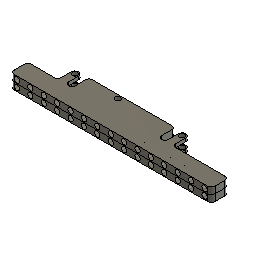
_Bottom Attatchment.85361469-475e-472e-92d3-0b1b0a94a3bd (Autodesk Fusion 360 design; units mm, degrees)
Autodesk Fusion 360 part; units mm, degrees
sketch "Sketch1" plane through (0, 0, 0) normal (0, 1, 0) x (1, 0, 0)
  circle A0 centre (25.25, 23) radius 2
  circle A1 centre (57.25, 23) radius 2
  circle A2 centre (105.25, 23) radius 2
  circle A3 centre (25.25, 23) radius 2.75
  circle A4 centre (57.25, 23) radius 2.75
  circle A5 centre (105.25, 23) radius 2.75
  line L0 (28, 23) -> (28, 13)
  line L1 (28, 13) -> (33, 13)
  line L2 (33, 13) -> (33, 25.75)
  line L3 (33, 25.75) -> (97.5, 25.75)
  line L4 (97.5, 25.75) -> (97.5, 13)
  line L5 (97.5, 13) -> (102.5, 13)
  line L6 (102.5, 13) -> (102.5, 23)
  line L7 (108, 23) -> (108, 13)
  line L8 (108, 13) -> (150, 13)
  line L9 (150, 13) -> (150, 0)
  line L10 (150, 0) -> (0, 0)
  line L11 (0, 0) -> (0, 13)
  line L12 (0, 13) -> (22.5, 13)
  line L13 (22.5, 13) -> (22.5, 23)
  line L14 (25.25, 25.75) -> (15.4724, 25.75)
  line L15 (105.25, 25.75) -> (113, 25.75)
  line L16 (108, 13) -> (102.5, 13)
  line L17 (28, 13) -> (22.5, 13)
  line L18 (33, 0) -> (97.5, 0) construction
  line L19 (97.5, 0) -> (97.5, 13) construction
  line L20 (97.5, 13) -> (33, 13) construction
  line L21 (33, 13) -> (33, 0) construction
  dimension "d1" = 4
  dimension "d2" = 5.5
  dimension "d3" = 32
  dimension "d4" = 80
  dimension "d5" = 10
  dimension "d6" = 5
  dimension "d7" = 23
  dimension "d8" = 22.5
  dimension "d9" = 42
  dimension "d10" = 10
  dimension "d33" = 150
  constraint equal A0 A1
  constraint equal A1 A2
  constraint concentric A0 A3
  constraint concentric A1 A4
  constraint concentric A2 A5
  constraint equal A4 A5
  constraint equal A3 A4
  constraint coincident A3 L0.start
  constraint vertical L0
  constraint perpendicular L0 L1
  constraint perpendicular L1 L2
  constraint perpendicular L2 L3
  constraint perpendicular L3 L4
  constraint perpendicular L2 L5
  constraint coincident A5 L6.end
  constraint tangent A5 L6
  constraint coincident A5 L7.start
  constraint parallel L6 L7
  constraint perpendicular L8 L9
  constraint coincident L10.end L11.start
  constraint perpendicular L10 L11
  constraint perpendicular L9 L12
  constraint coincident A3 L13.end
  constraint tangent A3 L13
  constraint horizontal L10
  constraint horizontal L12
  constraint vertical L13
  constraint tangent A4 L3
  constraint coincident A3 L14.start
  constraint horizontal L14
  constraint coincident A5 L15.start
  constraint horizontal L15
  constraint tangent A5 L15
  constraint tangent A3 L14
  constraint collinear L3 L14
  constraint collinear L3 L15
  constraint vertical L6
  constraint equal L7 L13
  constraint equal L1 L5
  constraint equal L2 L4
  constraint equal L6 L7
  constraint tangent A5 L7
  constraint tangent A3 L0
  constraint coincident L10
  constraint coincident L1.end
  constraint collinear L4 L19
  measures "d1" diameter of A0
  measures "d2" diameter of A3
  measures "d3" distance of A0.centre A1.centre
  measures "d4" distance of A0.centre A2.centre
  measures "d5" distance of L7.start L7.end
  measures "d6" distance of L4.end L5.end
  measures "d7" distance of A0.centre L10
  measures "d8" distance of L11.end L12.end
  measures "d9" distance of L7.end L8.end
  measures "d33" distance of L9.end L10.end
extrude "Extrude1" add sketch "Sketch1" along normal blind 5 contours A4 | L1 L2 L3 L4 L5 L8 L9 L10 L11 L12 L16 L17 makes body 1
extrude "Extrude2" add sketch "Sketch1" along normal blind 5 and the other way blind -2.5 contours A3 | A3 L0 L13 L17 | A5 L6 L7 L16 | A5 bodies 1
fillet "Fillet1" radius 2.5 8 edges at (33, 2.5, -25.75) (97.5, 2.5, -25.75) (102.5, 3.75, -13) (97.5, 2.5, -13) (108, 3.75, -13) (33, 2.5, -13) (28, 3.75, -13) (22.5, 3.75, -13) on bodies 1
fillet "Fillet1" radius 3 4 edges at (0, 2.5, -13) (0, 2.5, 0) (150, 2.5, 0) (150, 2.5, -13) on bodies 1
sketch "Sketch2" plane through (0, 0, 0) normal (0, 0, 1) x (1, 0, 0)
  line L0 (147, 0) -> (147, 5)
  line L1 (147, 5) -> (3, 5)
  line L2 (3, 5) -> (3, 0)
  line L3 (3, 0) -> (147, 0)
  circle A0 centre (5, 2.5) radius 1.95
  line L4 (0, 5) -> (0, 0)
  line L5 (5, 2.5) -> (3, 2.5)
  dimension "d25" = 5
  dimension "d26" = 3.9
  constraint midpoint L2 L5.end
  constraint perpendicular L2 L5
  constraint coincident A0.centre L5.start
  measures "d25" distance of A0.centre L4
  measures "d26" diameter of A0
extrude "Extrude4" cut sketch "Sketch2" against normal blind 5 contours A0 bodies 1
pattern_linear "R-Pattern1" count 15 spacing 10 along (1, 0, 0) of "Extrude4"
mirror "Mirror1" about plane through (0, 0, 0) normal (0, 1, 0) of bodies 1 makes body 2
equation "d15 = -5 mm + 2.5 mm"
named bodies: "BottomAttatchR", "BottomAttatchL"
